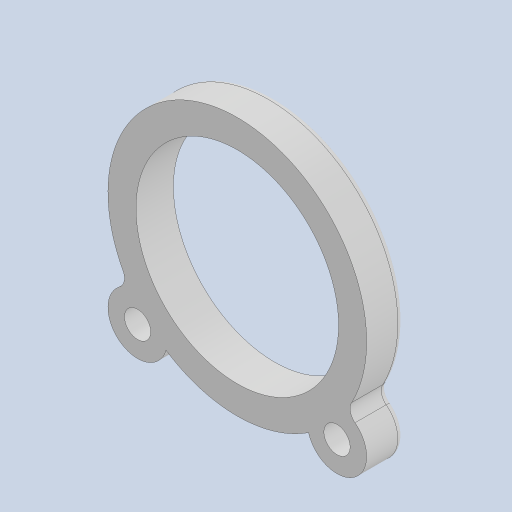
# Autodesk Inventor part: cage_inside_07
Saved by Autodesk Inventor 2024.4 (Build 284460030, 460C)
## iProperties
Created: 2026-07-27
Part Number: cage_inside_07
Material: Generic
Document SubType Name: Modeling
Designer: tooles01
Density: 1 g/cm^3
Appearance: Default
Author: tooles01
Autodesk Inventor part; units mm, degrees
ref_plane "YZ Plane" through (0, 0, 0) normal (1, 0, 0) x (0, 1, 0)
ref_plane "XZ Plane" through (0, 0, 0) normal (0, 1, 0) x (-1, 0, 0)
sketch "Sketch1: base" plane through (0, 0, 0) normal (0, 0, 1) x (1, 0, 0)
  circle A0 centre (-5, 4) radius 16.25
  circle A1 centre (-5, 4) radius 20.75
  circle A2 centre (-21, -12) radius 4.75
  circle A3 centre (11, -12) radius 4.75
  line L0 (-21, -12) -> (11, -12) construction
  line L1 (-21, 20) -> (-21, -12) construction
  point P0 (0, 0)
  point P1 (-5, -12)
  point P2 (-21, 4)
  point P3 (-22.3145, -7.4355)
  point P4 (-16.4355, -13.3145)
  point P5 (6.4355, -13.3145)
  point P6 (12.3145, -7.4355)
  dimension "d0" = 9.5
  dimension "d1" = 32
  dimension "d2" = 41.5
  dimension "d3" = 32.5
  dimension "d4" = 32
  constraints: 4 centre point, 4 end point, 3 coincident, 2 midpoint, 1 equal radius, 1 horizontal, 1 horizontal alignment, 1 perpendicular, 1 vertical alignment, 1 other
  measures "d0" diameter of A2
  measures "d1" distance of L0.start L0.end
  measures "d2" diameter of A1
  measures "d3" diameter of A0
  measures "d4" distance of L1.start L0.start
sketch "Sketch2: tube stopper" plane through (0, 0, 0) normal (0, 0, 1) x (1, 0, 0)
  circle A0 centre (-5, 4) radius 14.875
  circle A1 centre (-5, 4) radius 16.25 projected
  point P0 (0, 0)
  dimension "d14" = 29.75
  constraints: 1 centre point, 1 coincident
  measures "d14" diameter of A0
extrude "Ex1: base" add sketch "Sketch1: base" along normal blind 6
ref_plane "Work Plane2" through (0, 0, 0) normal (0, 0, 1) x (1, 0, 0)
sketch "Sketch: text" plane through (0, 0, 0) normal (0, 0, -1) x (-1, 0, 0)
  line L0 (3.25, 23.8) -> (6.75, 23.8) construction
  line L1 (6.75, 23.8) -> (6.75, 20.3) construction
  line L2 (6.75, 20.3) -> (3.25, 20.3) construction
  line L3 (3.25, 20.3) -> (3.25, 23.8) construction
  line L4 (2.1748, 22.7624) -> (3.0901, 22.7624)
  line L5 (3.0901, 22.7624) -> (3.5386, 21.3071)
  line L6 (3.5386, 21.3071) -> (3.9993, 22.7624)
  line L7 (3.9993, 22.7624) -> (4.8871, 22.7624)
  line L8 (4.8871, 22.7624) -> (3.9108, 20.465)
  line L9 (3.9108, 20.465) -> (3.1297, 20.465)
  line L10 (3.1297, 20.465) -> (2.1748, 22.7624)
  line L11 (5.0732, 23.635) -> (7.6422, 23.635)
  line L12 (7.6422, 23.635) -> (7.6422, 23.0401)
  spline S0 degree 2 poles (7.6422, 23.0401) (7.3066, 22.738) (7.0838, 22.3841) knots 0 0 0 1 1 1
  spline S1 degree 2 poles (7.0838, 22.3841) (6.8123, 21.9569) (6.6536, 21.4322) knots 0 0 0 1 1 1
  spline S2 degree 2 poles (6.6536, 21.4322) (6.5286, 21.0233) (6.4858, 20.465) knots 0 0 0 1 1 1
  line L13 (6.4858, 20.465) -> (5.6072, 20.465)
  spline S3 degree 2 poles (5.6072, 20.465) (5.7109, 21.24) (6.1563, 22.2926) (6.6384, 22.8906) knots 0 0 0 1 2 2 2
  line L14 (6.6384, 22.8906) -> (5.0732, 22.8906)
  line L15 (5.0732, 22.8906) -> (5.0732, 23.635)
  point P0 (0, 0)
  point P1 (5, 4)
  point P2 (5, 20.3)
  dimension "d22" = 3.5
  dimension "d23" = 16.3
  constraints: 1 midpoint, 1 perpendicular, 1 vertical, 1 vertical alignment, 2 other
  measures "d22" distance of L0.start L0.end
  measures "d23" distance from line of point (5, 4) L2
hole "Hole1: M3 heat-sets" at (11, -12, 0) at (-21, -12, 0) direction (0, 0, -1) diameter 4.2 end through all both
extrude "Ex: tube stopper" [suppressed]
fillet "Fillet1" radius 2 2 edges at (12.3145, -7.4355, 3) (-22.3145, -7.4355, 3)
fillet "Fillet2" radius 1 5 edges at (-23.1529, -7.0697, 0) (-23.6764, -15.9242, 0) (13.1529, -7.0697, 0) (13.6764, -15.9242, 0) (-5, 24.75, 0)
extrude "Ex: text" cut sketch "Sketch: text" against normal blind 1 from surface at 0
body "Solid1"
